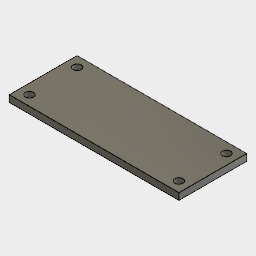
Switch Plate_ CSA011040∩╗┐ (Autodesk Fusion 360 design; units mm, degrees)
Autodesk Fusion 360 part; units mm, degrees
sketch "Sketch1" plane through (0, 0, 0) normal (0, 1, 0) x (1, 0, 0) in component "Base Plate"
  line L0 (-125, 50) -> (125, 50)
  line L1 (125, 50) -> (125, -50)
  line L2 (125, -50) -> (-125, -50)
  line L3 (-125, -50) -> (-125, 50)
  line L4 (-125, 50) -> (125, -50) construction
  line L5 (125, 50) -> (-125, -50) construction
  circle A0 centre (-110, 35) radius 6
  circle A1 centre (-110, -35) radius 6
  line L6 (0, 0) -> (0, 50) construction
  circle A2 centre (110, 35) radius 6
  circle A3 centre (110, -35) radius 6
  dimension "d1" = 100
  dimension "d2" = 250
  dimension "d3" = 15
  dimension "d4" = 15
  dimension "d5" = 12
  dimension "d6" = 15
  measures "d1" distance of L0.end L1.end
  measures "d2" distance of L1.end L2.end
  measures "d3" distance of L0 A0.centre
  measures "d4" distance of L3 A0.centre
  measures "d5" diameter of A0
  measures "d6" distance of L2 A1.centre
extrude "Extrude1" add sketch "Sketch1" against normal blind 10 in component "Base Plate"
component "Base Plate" placed x (1, 0, 0) y (0, 1, 0) z (0, 0, 1) at (0, 0, 0)
